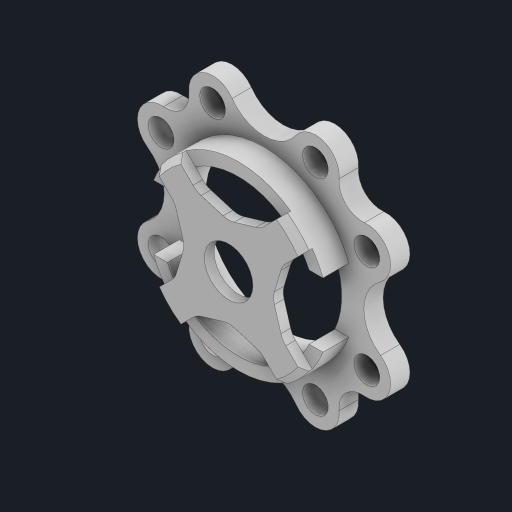
# Autodesk Inventor part: PotentiometerCover
Saved by Autodesk Inventor 2023 (Build 270158000, 158)
## iProperties
Created: 2023-07-17
Part Number: PotentiometerCover
Material: Generic
Document SubType Name: Modeling
Designer: valer
Density: 1 g/cm^3
Appearance: Default
Author: valer
Autodesk Inventor part; units mm, degrees
ref_plane "YZ Plane" through (0, 0, 0) normal (1, 0, 0) x (0, 1, 0)
ref_plane "XZ Plane" through (0, 0, 0) normal (0, 1, 0) x (-1, 0, 0)
ref_plane "XY Plane" through (0, 0, 0) normal (0, 0, 1) x (1, 0, 0)
sketch "Base" plane through (0, 0, 0) normal (0, 0, 1) x (1, 0, 0)
  arc A0 (-3.0057, -11.8072) -> (-3.0057, -19.8072) centre (-14.3194, -15.8072) ccw construction
  circle A1 centre (-14.3194, -15.8072) radius 3.775 projected
  circle A2 centre (-14.3194, -15.8072) radius 12.09
  circle A3 centre (-14.3194, -15.8072) radius 14.09
  point P0 (0, 0)
  dimension "d1" = 12
  dimension "d2" = 24.18
  dimension "d3" = 2
  constraints: 2 centre point, 2 coincident
  measures "d1" radius of A0
  measures "d2" diameter of A2
  measures "d3" radial gap between concentric circles of A2 A3
extrude "BaseFeature" add sketch "Base" along normal blind 1.5 contours A2 | A3
sketch "Head" plane through (-14.3194, -15.8072, 0) normal (0, 0, -1) x (-1, 0, 0)
  circle A0 centre (0, 0) radius 14.09 projected
  circle A1 centre (0, 0) radius 12.09 projected
  point P0 (-14.3194, 15.8072)
extrude "HeadFeature" add sketch "Head" along normal blind 7
sketch "Mount" plane through (-14.3194, -15.8072, -7) normal (0, 0, -1) x (-1, 0, 0)
  line L0 (-24, 24) -> (24, 24) construction
  line L1 (24, 24) -> (24, -24) construction
  line L2 (24, -24) -> (-24, -24) construction
  line L3 (-24, -24) -> (-24, 24) construction
  line L4 (0, 24) -> (0, -24) construction
  line L5 (-24, 0) -> (24, 0) construction
  circle A0 centre (0, 0) radius 7
  circle A1 centre (0, 0) radius 12 construction
  line L6 (0, 12) -> (-12, 0) construction
  line L7 (-12, 0) -> (0, -12) construction
  line L8 (0, -12) -> (12, 0) construction
  line L9 (12, 0) -> (0, 12) construction
  line L10 (-24, 16) -> (24, 16) construction
  line L11 (-24, 8) -> (24, 8) construction
  line L12 (-24, -8) -> (24, -8) construction
  line L13 (-24, -16) -> (24, -16) construction
  line L14 (-16, 24) -> (-16, -24) construction
  line L15 (-8, 24) -> (-8, -24) construction
  line L16 (16, 24) -> (16, -24) construction
  line L17 (8, 24) -> (8, -24) construction
  circle A2 centre (-8, 16) radius 2
  circle A3 centre (-16, 8) radius 2
  circle A4 centre (8, 16) radius 2
  line L18 (24, 8) -> (-24, 8) construction
  circle A5 centre (16, 8) radius 2
  circle A6 centre (-16, -8) radius 2
  circle A7 centre (-8, -16) radius 2
  circle A8 centre (8, -16) radius 2
  circle A9 centre (16, -8) radius 2
  circle A10 centre (0, 0) radius 14.09 projected
  circle A11 centre (0, 0) radius 21.59
  circle A12 centre (0, 0) radius 14.09 projected
  point P0 (-14.3194, 15.8072)
  dimension "d8" = 14
  dimension "d9" = 24
  dimension "d10" = 48
  dimension "d11" = 8
  dimension "d12" = 8
  dimension "d13" = 8
  dimension "d14" = 8
  dimension "d40" = 7.5
  constraints: 38 end point, 16 symmetric about line, 14 point on line, 11 centre point, 8 perpendicular, 5 midpoint, 4 coincident, 4 parallel, 2 point on circle, 1 horizontal, 6 other
  measures "d8" diameter of A0
  measures "d9" diameter of A1
  measures "d10" distance of L3.end L0.end
  measures "d11" distance between parallel lines of L0 L10
  measures "d12" distance between parallel lines of L11 L10
  measures "d13" distance between parallel lines of L3 L14
  measures "d14" distance between parallel lines of L14 L15
  measures "d40" radial gap between concentric circles of A11 A12
extrude "MountFeature" add sketch "Mount" against normal blind 3 contours A11
sketch "Cuts" plane through (-14.3194, -15.8072, 1.5) normal (0, 0, 1) x (1, 0, 0)
  circle A0 centre (0, 0) radius 14.09 projected
  line L0 (-11.4988, -8.1428) -> (-8.356, -5)
  line L1 (-8.356, -5) -> (-8.356, 5) construction
  line L2 (-8.356, 5) -> (-11.4988, 8.1428)
  line L3 (-8.356, 0) -> (-14.09, 0) construction
  line L4 (0, 0) -> (-21.59, 0) construction
  circle A1 centre (0, 0) radius 21.59 projected
  line L5 (0, 0) -> (0, -21.59) construction
  line L6 (-5, -8.356) -> (-8.1428, -11.4988)
  line L7 (-8.1428, -11.4988) -> (-11.4988, -8.1428) construction
  line L8 (0, 0) -> (-15.2664, -15.2664) construction
  circle A2 centre (-8, -16) radius 2 construction
  circle A3 centre (-16, -8) radius 2 construction
  line L9 (-8, -16) -> (-16, -8) construction
  line L10 (-5, -8.356) -> (-8.356, -5) construction
  line L11 (-5, 8.356) -> (-8.1428, 11.4988)
  line L12 (-8.356, -5) -> (-6.856, 0)
  line L13 (-8.356, 5) -> (-6.856, 0)
  line L14 (11.4988, -8.1428) -> (8.356, -5)
  line L15 (8.356, -5) -> (8.356, 5) construction
  line L16 (8.356, 5) -> (11.4988, 8.1428)
  line L17 (5, -8.356) -> (8.1428, -11.4988)
  line L18 (5, -8.356) -> (8.356, -5) construction
  line L19 (5, 8.356) -> (8.1428, 11.4988)
  line L20 (8.356, -5) -> (6.856, 0)
  line L21 (8.356, 5) -> (6.856, 0)
  line L22 (5, -8.356) -> (-5, -8.356) construction
  line L23 (5, 8.356) -> (-5, 8.356) construction
  line L24 (5, -8.356) -> (0, -6.856)
  line L25 (-5, -8.356) -> (0, -6.856)
  line L26 (5, 8.356) -> (0, 6.856)
  line L27 (0, 6.856) -> (-5, 8.356)
  point P0 (14.3194, 15.8072)
  point P1 (-12, -12)
  point P2 (-6.678, -6.678)
  point P3 (8.1428, 11.4988)
  point P4 (-8.1428, 11.4988)
  point P5 (8.1428, -11.4988)
  point P6 (11.4988, -8.1428)
  point P7 (11.4988, 8.1428)
  dimension "d20" = 45
  dimension "d22" = 45
  dimension "d23" = 10
  dimension "d24" = 45
  dimension "d26" = 1.5
  dimension "d27" = 1.5
  dimension "d28" = 1.5
  constraints: 56 end point, 11 symmetric about line, 7 point on circle, 4 horizontal, 4 point on line, 3 midpoint, 2 vertical, 1 collinear, 1 equal length, 1 perpendicular
  measures "d20" angle of L3 L2
  measures "d22" angle of L0 L3
  measures "d23" distance of L0.end L1.end
  measures "d24" angle of L6 L5
  measures "d26" distance from line of L1 L12.end
  measures "d27" distance from line of L22 L24.end
  measures "d28" distance from line of L23 L26.end
extrude "CutsFeature" cut sketch "Cuts" against normal blind 1.5 contours A0 L14 L20 L21 L16 | L19 L26 L27 L11 A0 | A0 L6 L25 L24 L17 | L2 L13 L12 L0 A0
chamfer "CutsChamferFeature" distance 1 angle 45 4 edges at (-4.3563, -5.8441, 1.5) (-4.3563, -25.7704, 1.5) (-24.2826, -5.8441, 1.5) (-24.2826, -25.7704, 1.5)
fillet "CutsFilletFeature" radius 3 12 edges at (-5.9635, -10.8072, 0.75) (-7.4635, -15.8072, 0.75) (-5.9635, -20.8072, 0.75) (-22.6754, -10.8072, 0.75) (-21.1754, -15.8072, 0.75) (-22.6754, -20.8072, 0.75) (-19.3194, -24.1632, 0.75) (-14.3194, -22.6632, 0.75) (-9.3194, -24.1632, 0.75) (-19.3194, -7.4513, 0.75) (-14.3194, -8.9513, 0.75) (-9.3194, -7.4513, 0.75)
sketch "LeadCut" plane through (-14.3194, -15.8072, 0) normal (0, 0, 1) x (1, 0, 0)
  line L0 (11.0076, -5) -> (14.09, -5)
  line L1 (14.09, -5) -> (14.09, 5)
  line L2 (14.09, 5) -> (11.0076, 5)
  line L3 (11.0076, 5) -> (11.0076, -5)
  line L4 (0, 0) -> (21.59, 0) construction
  circle A0 centre (0, 0) radius 21.59 projected
  arc A1 (10.0606, -6.7046) -> (10.0606, 6.7046) centre (0, 0) ccw construction
  arc A2 (11.4988, -8.1428) -> (11.4988, 8.1428) centre (0, 0) ccw construction
  circle A3 centre (0, 0) radius 3.775 projected
  line L5 (0, 0) -> (0, 21.59) construction
  line L6 (-11.0076, -5) -> (-14.09, -5)
  line L7 (-14.09, -5) -> (-14.09, 5)
  line L8 (-14.09, 5) -> (-11.0076, 5)
  line L9 (-11.0076, 5) -> (-11.0076, -5)
  point P0 (14.3194, 15.8072)
  point P1 (14.09, 0)
  dimension "d35" = 10
  constraints: 20 end point, 4 point on circle, 4 symmetric about line, 2 horizontal, 2 parallel, 1 coincident, 1 midpoint, 1 perpendicular, 1 point on line, 1 vertical
  measures "d35" distance of L0.end L1.end
extrude "LeadCutFeature" cut sketch "LeadCut" against normal up to surface (4 mm away) contours L3 L2 L1 L0 | L6 L7 L8 L9
sketch "MountProfile" plane through (-14.3194, -15.8072, -4) normal (0, 0, 1) x (1, 0, 0)
  circle A0 centre (16, 8) radius 2 projected
  circle A1 centre (8, 16) radius 2 projected
  circle A2 centre (16, 8) radius 3.7015
  circle A3 centre (8, 16) radius 3.7015
  circle A4 centre (0, 0) radius 21.59 projected
  circle A5 centre (16, 8) radius 2 projected
  line L0 (16, 8) -> (8, 16) construction
  circle A6 centre (0, 0) radius 3.775 projected
  line L1 (0, 0) -> (12, 12) construction
  circle A7 centre (0, 0) radius 21.59 projected
  arc A8 (11.6827, 15.6282) -> (15.6282, 11.6827) centre (15.2664, 15.2664) ccw
  line L2 (0, 0) -> (-15.2664, 15.2664) construction
  line L3 (0, 0) -> (0, 21.59) construction
  circle A9 centre (-8, 16) radius 2 projected
  circle A10 centre (-16, 8) radius 2 projected
  circle A11 centre (-8, 16) radius 3.7015
  circle A12 centre (-16, 8) radius 3.7015
  arc A13 (-15.6282, 11.6827) -> (-11.6827, 15.6282) centre (-15.2664, 15.2664) ccw
  line L4 (0, 0) -> (-21.59, 0) construction
  circle A14 centre (16, -8) radius 3.7015
  circle A15 centre (8, -16) radius 3.7015
  arc A16 (15.6282, -11.6827) -> (11.6827, -15.6282) centre (15.2664, -15.2664) ccw
  circle A17 centre (-8, -16) radius 3.7015
  circle A18 centre (-16, -8) radius 3.7015
  arc A19 (-11.6827, -15.6282) -> (-15.6282, -11.6827) centre (-15.2664, -15.2664) ccw
  circle A20 centre (0, -21.59) radius 6.0581
  circle A21 centre (0, 21.59) radius 6.0581
  arc A22 (18.1201, 4.9659) -> (18.1201, -4.9659) centre (21.59, 0) ccw
  arc A23 (-18.1201, -4.9659) -> (-18.1201, 4.9659) centre (-21.59, 0) ccw
  point P0 (14.3194, 15.8072)
  point P1 (-9.6553, -19.3107)
  point P2 (-19.3107, -9.6553)
  point P3 (-9.6553, 19.3107)
  point P4 (-19.3107, 9.6553)
  point P5 (19.3107, 9.6553)
  point P6 (9.6553, 19.3107)
  point P7 (19.3107, -9.6553)
  point P8 (9.6553, -19.3107)
  point P9 (5.9981, 20.7401)
  point P10 (4.9659, 18.1201)
  point P11 (-4.9659, 18.1201)
  point P12 (-5.9981, 20.7401)
  point P13 (4.9659, -18.1201)
  point P14 (5.9981, -20.7401)
  point P15 (-5.9981, -20.7401)
  point P16 (-4.9659, -18.1201)
  constraints: 26 point on circle, 12 centre point, 10 end point, 10 symmetric about line, 7 coincident, 6 tangent, 3 horizontal, 1 equal radius, 1 midpoint, 1 perpendicular, 1 vertical, 22 other
extrude "MountProfileFeature" cut sketch "MountProfile" against normal through all contours A8 A3 A4 A2 | A2 A4 A14 A22 | A3 A21 A4 | A21 A4 | A14 A4 A15 A16 | A4 A21 | A11 A4 A21 | A4 A20 A15 | A11 A13 A12 A4 | A20 A4 | A20 A4 | A12 A23 A18 A4 | A20 A4 A17 | A18 A19 A17 A4
equation "\"d22\" = d20"
equation "\"d24\" = d20"
equation "\"d27\" = d26"
equation "\"d28\" = d26"
body "Solid1"
